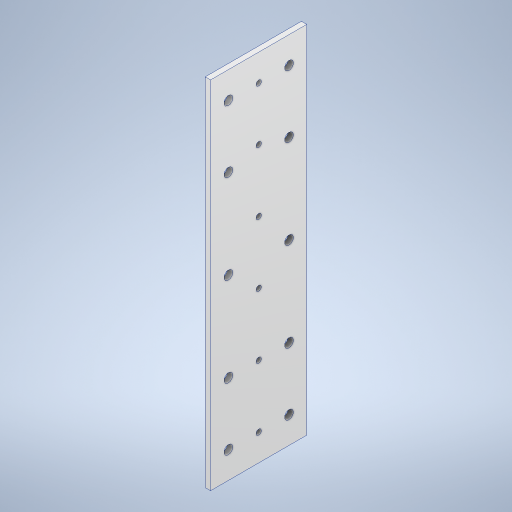
# Autodesk Inventor part: linrail_fix
Saved by Autodesk Inventor 2024 (Build 280153000, 153)
## iProperties
Created: 2025-12-26
Part Number: linrail_fix
Material: Aluminum 6061
Document SubType Name: Modeling
Designer: schar
Density: 2.7 g/cm^3
Appearance: Aluminum - Flat
Author: schar
Autodesk Inventor part; units mm, degrees
ref_plane "YZ Plane" through (0, 0, 0) normal (1, 0, 0) x (0, 1, 0)
ref_plane "XZ Plane" through (0, 0, 0) normal (0, 1, 0) x (-1, 0, 0)
ref_plane "XY Plane" through (0, 0, 0) normal (0, 0, 1) x (1, 0, 0)
sketch "Sketch1" plane through (0, 0, 0) normal (1, 0, 0) x (0, 1, 0)
  line L0 (0, 0) -> (-200, 0)
  line L1 (-200, 0) -> (-200, -54.112)
  line L2 (-200, -54.112) -> (0, -54.112)
  line L3 (0, -54.112) -> (0, 0)
  line L4 (0, -27.056) -> (-15, -27.056)
  line L5 (-15, -27.056) -> (-45, -27.056)
  line L6 (-45, -27.056) -> (-80, -27.056)
  line L7 (-80, -27.056) -> (-115, -27.056)
  line L8 (-115, -27.056) -> (-150, -27.056)
  line L9 (-150, -27.056) -> (-185, -27.056)
  circle A0 centre (-15, -27.056) radius 1.5
  circle A1 centre (-45, -27.056) radius 1.5
  circle A2 centre (-80, -27.056) radius 1.5
  circle A3 centre (-115, -27.056) radius 1.5
  circle A4 centre (-150, -27.056) radius 1.5
  circle A5 centre (-185, -27.056) radius 1.5
  dimension "d0" = 200
  dimension "d1" = 54.112
  dimension "d2" = 15
  dimension "d3" = 30
  dimension "d8" = 35
  dimension "d9" = 35
  dimension "d10" = 35
  dimension "d11" = 35
  dimension "d12" = 3
  dimension "d13" = 3
  dimension "d16" = 35
  constraints: 20 end point, 6 centre point, 4 horizontal, 4 point on line, 2 coincident, 2 parallel, 1 midpoint, 1 perpendicular, 8 other
  measures "d0" distance of L2.end L1.end
  measures "d1" distance of L1.end L0.end
  measures "d2" distance of L4.start L4.end
  measures "d3" distance of L4.end L5.end
  measures "d8" distance of L5.end L6.end
  measures "d9" distance of L6.end L7.end
  measures "d10" distance of L7.end L8.end
  measures "d11" distance of L8.end L9.end
  measures "d12" diameter of A0
  measures "d13" diameter of A1
  measures "d16" distance of A1.centre A2.centre
extrude "Extrusion1" add sketch "Sketch1" along normal blind 3
sketch "Sketch2" plane through (3, 0, 0) normal (1, 0, 0) x (0, 0, -1)
  line L0 (0, 0) -> (0, -200) projected
  line L1 (0, 0) -> (10, 0)
  line L2 (54.112, 0) -> (0, 0) projected
  line L3 (0, 0) -> (0, -50)
  line L4 (0, -50) -> (0, -100)
  line L5 (0, -100) -> (0, -150)
  line L6 (0, -150) -> (10, -150)
  line L7 (0, -50) -> (0, -15)
  line L8 (0, -15) -> (10, -15)
  line L9 (0, -50) -> (10, -50)
  line L10 (27.056, 0) -> (27.056, -7.4996)
  line L11 (0, -150) -> (0, -185)
  line L12 (0, -185) -> (10, -185)
  circle A0 centre (10, -185) radius 2.5
  circle A1 centre (10, -150) radius 2.5
  circle A2 centre (10, -100) radius 2.5
  circle A3 centre (10, -50) radius 2.5
  circle A4 centre (10, -15) radius 2.5
  circle A5 centre (44.112, -185) radius 2.5
  circle A6 centre (44.112, -150) radius 2.5
  circle A7 centre (44.112, -100) radius 2.5
  circle A8 centre (44.112, -50) radius 2.5
  circle A9 centre (44.112, -15) radius 2.5
  dimension "d23" = 10
  dimension "d24" = 50
  dimension "d25" = 50
  dimension "d26" = 50
  dimension "d27" = 35
  dimension "d28" = 35
  dimension "d29" = 5
  dimension "d30" = 5
  dimension "d33" = 50
  dimension "d38" = 5
  constraints: 22 end point, 10 centre point, 5 point on line, 5 symmetric about line, 3 coincident, 3 perpendicular, 2 midpoint, 2 vertical, 1 horizontal, 9 other
  measures "d23" distance of L0.start L1.end
  measures "d24" distance of L0.start L3.end
  measures "d25" distance of L3.end L4.end
  measures "d26" distance of L4.end L5.end
  measures "d27" distance of L3.end L7.end
  measures "d28" distance of L5.end L11.end
  measures "d29" diameter of A0
  measures "d30" diameter of A1
  measures "d33" distance of A1.centre A2.centre
  measures "d38" diameter of A4
extrude "Extrusion2" cut sketch "Sketch2" against normal blind 3
body "Solid1"
